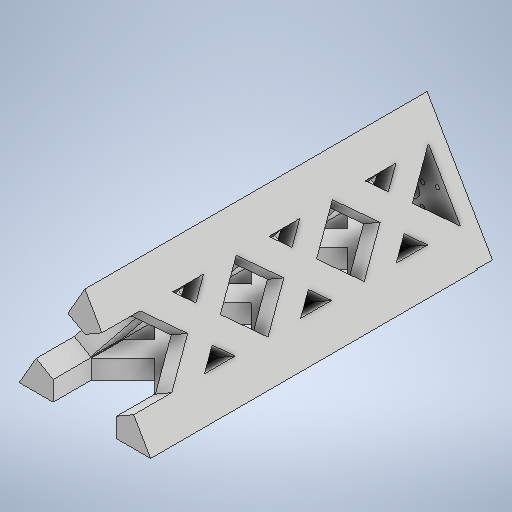
# Autodesk Inventor part: ChloeCallsThisTheEffielTower
Saved by Autodesk Inventor 2027 (Build 310192060, 192F)
## iProperties
Created: 2026-07-08
Part Number: ChloeCallsThisTheEffielTower
Material: Generic
Document SubType Name: Modeling
Designer: 13129
Density: 1 g/cm^3
Appearance: Default
Author: 13129
Autodesk Inventor part; units mm, degrees
ref_plane "YZ Plane" through (0, 0, 0) normal (1, 0, 0) x (0, 1, 0)
ref_plane "XZ Plane" through (0, 0, 0) normal (0, 1, 0) x (-1, 0, 0)
ref_plane "XY Plane" through (0, 0, 0) normal (0, 0, 1) x (1, 0, 0)
sketch "Sketch1" plane through (0, 0, 0) normal (0, 0, 1) x (1, 0, 0)
  line L0 (0, 0) -> (101.6, 0)
  line L1 (101.6, 0) -> (50.8, 87.9882)
  line L2 (0, 0) -> (50.8, 87.9882)
  dimension "d0" = 101.6
  dimension "d2" = 60
  constraints: 6 end point, 1 equal length, 1 horizontal
  measures "d0" distance of L0.start L0.end
  measures "d2" angle of L1 L0
extrude "Extrusion1" add sketch "Sketch1" along normal blind 12
sketch "Sketch2" plane through (0, 0, 12) normal (0, 0, 1) x (1, 0, 0)
  line L0 (101.6, 0) -> (50.8, 87.9882) construction
  line L1 (0, 0) -> (101.6, 0) construction
  line L2 (26.38, 43.9941) -> (75.22, 43.9941) construction
  line L3 (75.22, 43.9941) -> (75.22, 13.9941) construction
  line L4 (75.22, 13.9941) -> (26.38, 13.9941) construction
  line L5 (26.38, 13.9941) -> (26.38, 43.9941) construction
  circle A0 centre (50.8, 28.9941) radius 6.25
  circle A1 centre (42.3, 37.4941) radius 1.7
  circle A2 centre (42.3, 20.4941) radius 1.7
  circle A3 centre (59.3, 20.4941) radius 1.7
  circle A4 centre (59.3, 37.4941) radius 1.7
  circle A5 centre (70.8, 39.4941) radius 1.7
  circle A6 centre (70.8, 18.4941) radius 1.7
  circle A7 centre (30.8, 18.4941) radius 1.7
  circle A8 centre (30.8, 39.4941) radius 1.7
  line L6 (30.8, 39.4941) -> (70.8, 39.4941) construction
  line L7 (70.8, 39.4941) -> (70.8, 18.4941) construction
  line L8 (42.3, 37.4941) -> (59.3, 37.4941) construction
  line L9 (59.3, 37.4941) -> (59.3, 20.4941) construction
  point P0 (50.8, 13.9941)
  point P1 (50.8, 0)
  point P2 (76.2, 43.9941)
  point P3 (26.38, 28.9941)
  point P4 (50.8, 43.9941)
  point P5 (59.3, 28.9941)
  point P6 (75.22, 28.9941)
  point P7 (50.8, 37.4941)
  point P8 (50.8, 39.4941)
  point P9 (70.8, 28.9941)
  dimension "d5" = 48.84
  dimension "d6" = 30
  dimension "d7" = 12.5
  dimension "d8" = 3.4
  dimension "d9" = 17
  dimension "d10" = 17
  dimension "d11" = 40
  dimension "d12" = 21
  constraints: 16 end point, 10 midpoint, 9 centre point, 8 horizontal alignment, 8 vertical alignment, 7 equal radius, 3 horizontal, 3 perpendicular, 2 parallel
  measures "d5" distance of L3.end L4.end
  measures "d6" distance of L2.end L3.end
  measures "d7" diameter of A0
  measures "d8" diameter of A4
  measures "d9" distance of L8.start L8.end
  measures "d10" distance of L8.end L9.end
  measures "d11" distance of L6.start L6.end
  measures "d12" distance of L6.end L7.end
extrude "Extrusion2" cut sketch "Sketch2" against normal through all
sketch "Sketch3" plane through (0, 0, 12) normal (0, 0, 1) x (1, 0, 0)
  circle A0 centre (50.8, 28.9941) radius 6.25 construction
  line L0 (101.6, 0) -> (50.8, 87.9882) construction
  line L1 (50.8, 87.9882) -> (0, 0) construction
  line L2 (50.8, 57.5082) -> (37.6018, 65.1282)
  line L3 (50.8, 57.5082) -> (63.9982, 65.1282)
  line L4 (37.6018, 65.1282) -> (50.8, 87.9882)
  line L5 (63.9982, 65.1282) -> (50.8, 87.9882)
  line L6 (26.1061, 14.737) -> (26.1061, -0.503)
  line L7 (26.1061, 14.737) -> (12.9078, 22.357)
  line L8 (26.1061, -0.503) -> (-0.2904, -0.503)
  line L9 (12.9078, 22.357) -> (-0.2904, -0.503)
  line L10 (75.4939, 14.737) -> (88.6922, 22.357)
  line L11 (75.4939, 14.737) -> (75.4939, -0.503)
  line L12 (88.6922, 22.357) -> (101.8904, -0.503)
  line L13 (75.4939, -0.503) -> (101.8904, -0.503)
  dimension "d15" = 30.48
  dimension "d18" = 360
  constraints: 24 end point, 2 collinear, 2 perpendicular, 2 point on line, 1 vertical alignment, 25 other
  measures "d15" distance of L0.end L2.start
extrude "Extrusion3" add sketch "Sketch3" along normal blind 254
sketch "Sketch4" plane through (-0.2904, -0.503, 12) normal (0, -1, 0) x (1, 0, 0)
  line L0 (26.3965, 0) -> (26.3965, 254) construction
  line L1 (26.3965, 0) -> (75.7843, 49.3879)
  line L2 (75.7843, 0) -> (75.7843, 254) construction
  line L3 (26.3965, 0) -> (96.2414, 0) construction
  line L4 (26.3965, 25.4) -> (75.7843, 74.7879)
  line L5 (75.7843, 0) -> (26.3965, 49.3879)
  line L6 (26.3965, 0) -> (26.3965, 254) construction
  line L7 (75.7843, 0) -> (145.6293, 0) construction
  line L8 (75.7843, 25.4) -> (26.3965, 74.7879)
  line L9 (26.3965, 0) -> (26.3965, 254)
  line L10 (75.7843, 254) -> (75.7843, 0)
  line L11 (88.9825, 0) -> (64.2886, 0) construction
  line L12 (26.3965, 74.7879) -> (75.7843, 124.1757)
  line L13 (26.3965, 74.7879) -> (96.2414, 74.7879) construction
  line L14 (75.7843, 74.7879) -> (26.3965, 124.1757)
  line L15 (75.7843, 74.7879) -> (145.6293, 74.7879) construction
  line L16 (26.3965, 100.1879) -> (75.7843, 149.5757)
  line L17 (75.7843, 100.1879) -> (26.3965, 149.5757)
  line L18 (26.3965, 149.5757) -> (75.7843, 198.9636)
  line L19 (26.3965, 149.5757) -> (96.2414, 149.5757) construction
  line L20 (75.7843, 149.5757) -> (26.3965, 198.9636)
  line L21 (75.7843, 149.5757) -> (156.0868, 149.5757) construction
  line L22 (26.3965, 174.9757) -> (75.7843, 224.3636)
  line L23 (75.7843, 174.9757) -> (26.3965, 224.3636)
  point P0 (0.2904, -12)
  point P1 (51.0904, 199.6696)
  point P2 (38.3904, 186.9696)
  point P3 (51.0904, 174.2696)
  point P4 (63.7904, 186.9696)
  point P5 (51.0904, 124.8818)
  point P6 (38.3904, 112.1818)
  point P7 (26.3965, 74.7879)
  point P8 (26.3965, 74.7879)
  point P9 (51.0904, 99.4818)
  point P10 (75.7843, 74.7879)
  point P11 (75.7843, 74.7879)
  point P12 (63.7904, 112.1818)
  point P13 (38.3904, 37.3939)
  point P14 (51.0904, 24.6939)
  point P15 (63.7904, 37.3939)
  point P16 (51.0904, 50.0939)
  dimension "d22" = 45
  dimension "d23" = 25.4
  dimension "d24" = 135
  dimension "d25" = 25.4
  dimension "d26" = 45
  dimension "d27" = 135
  dimension "d28" = 25.4
  dimension "d29" = 25.4
  dimension "d30" = 45
  dimension "d31" = 135
  dimension "d32" = 25.4
  dimension "d33" = 25.4
  constraints: 40 end point, 18 point on line, 11 equal length, 6 horizontal, 2 perpendicular
  measures "d22" angle of L3 L1
  measures "d23" distance of L0.start L4.start
  measures "d24" angle of L7 L5
  measures "d25" distance of L8.start L2.start
  measures "d26" angle of L13 L12
  measures "d27" angle of L15 L14
  measures "d28" distance of L16.start L8.end
  measures "d29" distance of L4.end L17.start
  measures "d30" angle of L19 L18
  measures "d31" angle of L21 L20
  measures "d32" distance of L22.start L17.end
  measures "d33" distance of L16.end L23.start
extrude "Extrusion4" add sketch "Sketch4" against normal blind 14.732 contours L9 L4 L5 L1 | L5 L4 L8 L1 | L1 L8 L10 L5 | L8 L4 L10 L1 | L5 L9 L8 L4 | L9 L16 L14 L12 | L14 L12 L17 L10 | L14 L16 L17 L12 | L9 L17 L16 L14 | L17 L16 L10 L12 | L9 L22 L20 L18 | L20 L18 L23 L10 | L20 L22 L23 L18 | L9 L23 L22 L20 | L23 L22 L10 L18
sketch "Sketch5" plane through (50.8, 87.9882, 0) normal (-0.8660254, 0.5, 0) x (0, 0, 1)
  line L0 (12, -75.7843) -> (266, -75.7843) construction
  line L1 (12, -26.3965) -> (61.3879, -75.7843)
  line L2 (12, -26.3965) -> (81.845, -26.3965) construction
  line L3 (12, -75.7843) -> (61.3879, -26.3965)
  line L4 (12, -26.3965) -> (266, -26.3965) construction
  line L5 (12, -75.7843) -> (81.845, -75.7843) construction
  line L6 (37.4, -26.3965) -> (86.7879, -75.7843)
  line L7 (37.4, -75.7843) -> (86.7879, -26.3965)
  line L8 (12, -13.1982) -> (12, -26.3965) construction
  line L9 (12, -26.3965) -> (266, -26.3965)
  line L10 (12, -75.7843) -> (266, -75.7843)
  line L11 (86.7879, -26.3965) -> (136.1757, -75.7843)
  line L12 (86.7879, -26.3965) -> (148.6929, -26.3965) construction
  line L13 (86.7879, -75.7843) -> (136.1757, -26.3965)
  line L14 (86.7879, -75.7843) -> (156.6328, -75.7843) construction
  line L15 (112.1879, -26.3965) -> (161.5757, -75.7843)
  line L16 (112.1879, -75.7843) -> (161.5757, -26.3965)
  line L17 (161.5757, -26.3965) -> (210.9636, -75.7843)
  line L18 (161.5757, -26.3965) -> (231.4207, -26.3965) construction
  line L19 (161.5757, -75.7843) -> (210.9636, -26.3965)
  line L20 (161.5757, -75.7843) -> (231.4207, -75.7843) construction
  line L21 (186.9757, -26.3965) -> (236.3636, -75.7843)
  line L22 (186.9757, -75.7843) -> (236.3636, -26.3965)
  point P0 (198.9696, -63.7904)
  point P1 (211.6696, -51.0904)
  point P2 (236.3636, -26.3965)
  point P3 (198.9696, -38.3904)
  point P4 (186.2696, -51.0904)
  point P5 (124.1818, -63.7904)
  point P6 (136.8818, -51.0904)
  point P7 (124.1818, -38.3904)
  point P8 (111.4818, -51.0904)
  point P9 (49.3939, -63.7904)
  point P10 (62.0939, -51.0904)
  point P11 (49.3939, -38.3904)
  point P12 (36.6939, -51.0904)
  dimension "d36" = 45
  dimension "d37" = 45
  dimension "d38" = 25.4
  dimension "d39" = 25.4
  dimension "d40" = 45
  dimension "d41" = 45
  dimension "d42" = 25.4
  dimension "d43" = 25.4
  dimension "d44" = 45
  dimension "d45" = 45
  dimension "d46" = 25.4
  dimension "d47" = 25.4
  constraints: 40 end point, 18 point on line, 13 equal length, 6 horizontal
  measures "d36" angle of L1 L2
  measures "d37" angle of L5 L3
  measures "d38" distance of L1.start L6.start
  measures "d39" distance of L7.start L0.start
  measures "d40" angle of L11 L12
  measures "d41" angle of L14 L13
  measures "d42" distance of L7.end L15.start
  measures "d43" distance of L16.start L6.end
  measures "d44" angle of L17 L18
  measures "d45" angle of L20 L19
  measures "d46" distance of L21.end L17.end
  measures "d47" distance of L15.end L22.start
extrude "Extrusion5" add sketch "Sketch5" against normal blind 14.732 contours L9 L6 L3 L1 | L3 L6 L7 L1 | L1 L7 L10 L3 | L7 L6 L10 L1 | L3 L9 L7 L6 | L9 L15 L13 L11 | L13 L11 L16 L10 | L13 L15 L16 L11 | L9 L16 L15 L13 | L16 L15 L10 L11 | L9 L21 L19 L17 | L19 L17 L22 L10 | L19 L21 L22 L17 | L9 L22 L21 L19 | L22 L21 L10 L17
sketch "Sketch6" plane through (50.8, 87.9882, 266) normal (0.8660254, 0.5, 0) x (0, 0, -1)
  line L0 (0, -102.1808) -> (0, -75.7843) construction
  line L1 (254, -75.7843) -> (204.6121, -26.3965)
  line L2 (254, -26.3965) -> (0, -26.3965) construction
  line L3 (254, -75.7843) -> (323.845, -75.7843) construction
  line L4 (254, -75.7843) -> (0, -75.7843)
  line L5 (254, -26.3965) -> (0, -26.3965)
  line L6 (229.3061, -38.3035) -> (254, -25.9565) construction
  line L7 (254, -25.9565) -> (204.1722, -75.7843)
  line L8 (254, -75.7843) -> (0, -75.7843) construction
  line L9 (254, -25.9565) -> (324.4671, -25.9565) construction
  line L10 (228.6, -75.7843) -> (179.2121, -26.3965)
  line L11 (228.6, -26.3965) -> (179.2121, -75.7843)
  line L12 (179.2121, -26.3965) -> (129.8243, -75.7843)
  line L13 (179.2121, -26.3965) -> (249.0571, -26.3965) construction
  line L14 (179.2121, -75.7843) -> (129.8243, -26.3965)
  line L15 (179.2121, -75.7843) -> (249.0571, -75.7843) construction
  line L16 (153.8121, -75.7843) -> (104.4243, -26.3965)
  line L17 (104.4243, -75.7843) -> (153.8121, -26.3965)
  line L18 (153.8121, -25.9565) -> (179.2121, -25.9565) construction
  line L19 (104.4243, -75.7843) -> (55.0364, -26.3965)
  line L20 (104.4243, -75.7843) -> (174.2693, -75.7843) construction
  line L21 (104.4243, -26.3965) -> (55.0364, -75.7843)
  line L22 (104.4243, -26.3965) -> (174.2693, -26.3965) construction
  line L23 (79.0243, -75.7843) -> (29.6364, -26.3965)
  line L24 (29.6364, -75.7843) -> (79.0243, -26.3965)
  point P0 (266, -50.8)
  point P1 (54.3304, -51.0904)
  point P2 (29.6364, -75.7843)
  point P3 (67.0304, -63.7904)
  point P4 (79.7304, -51.0904)
  point P5 (67.0304, -38.3904)
  point P6 (129.1182, -51.0904)
  point P7 (141.8182, -63.7904)
  point P8 (154.5182, -51.0904)
  point P9 (141.8182, -38.3904)
  point P10 (203.9061, -51.0904)
  point P11 (204.1722, -75.7843)
  point P12 (216.3861, -63.5704)
  point P13 (229.0861, -50.8704)
  point P14 (253.5601, -26.3965)
  point P15 (216.6061, -38.3904)
  dimension "d50" = 135
  dimension "d51" = 135
  dimension "d52" = 25.4
  dimension "d53" = 25.4
  dimension "d54" = 135
  dimension "d55" = 135
  dimension "d56" = 25.4
  dimension "d57" = 25.4
  dimension "d58" = 135
  dimension "d59" = 135
  dimension "d60" = 25.4
  dimension "d61" = 25.4
  constraints: 38 end point, 7 horizontal, 6 equal length, 6 parallel, 1 perpendicular, 1 point on line, 21 other
  measures "d50" angle of L3 L1
  measures "d51" angle of L7 L9
  measures "d52" distance of L11.start L2.start
  measures "d53" distance of L10.start L1.start
  measures "d54" angle of L12 L13
  measures "d55" angle of L15 L14
  measures "d56" distance of L17.end L10.end
  measures "d57" distance of L16.start L11.end
  measures "d58" angle of L20 L19
  measures "d59" angle of L21 L22
  measures "d60" distance of L23.end L19.end
  measures "d61" distance of L24.start L21.end
extrude "Extrusion6" add sketch "Sketch6" against normal blind 14.732 contours L4 L10 L7 L1 | L7 L10 L11 L1 | L1 L11 L5 L7 | L11 L10 L5 L1 | L7 L4 L11 L10 | L4 L16 L12 L14 | L12 L14 L17 L5 | L12 L16 L17 L14 | L4 L17 L16 L12 | L17 L16 L5 L14 | L4 L23 L21 L19 | L21 L19 L24 L5 | L21 L23 L24 L19 | L4 L24 L23 L21 | L24 L23 L5 L19
body "Solid1"
